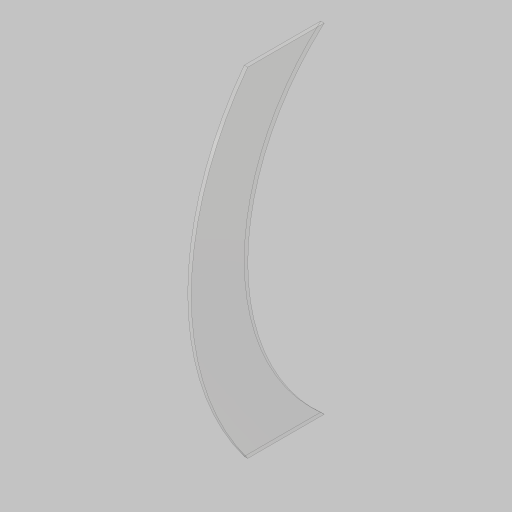
# Autodesk Inventor part: GP5-001
Saved by Autodesk Inventor 2023.5 (Build 275446000, 446)
## iProperties
Created: 2025-01-29
Part Number: GP5-001
Material: Polycarbonate, Clear
Document SubType Name: Sheet Metal
Designer: slick
Density: 1.2 g/cm^3
Sheet Metal Rule: Default
Appearance: Polycarbonate - Clear
Author: slick
Autodesk Inventor part; units mm, degrees
ref_plane "YZ Plane" through (0, 0, 0) normal (1, 0, 0) x (0, 1, 0)
ref_plane "XZ Plane" through (0, 0, 0) normal (0, 1, 0) x (-1, 0, 0)
ref_plane "XY Plane" through (0, 0, 0) normal (0, 0, 1) x (1, 0, 0)
sketch "Sketch1" plane through (0, 0, 0) normal (1, 0, 0) x (0, 1, 0)
  circle A0 centre (0, 0) radius 203.2 construction
  arc A1 (152.4, 134.4042) -> (-152.4, 134.4042) centre (0, 0) ccw
  arc A2 (152.4, 203.2) -> (-152.4, 203.2) centre (0, 0) ccw
  line L0 (152.4, 203.2) -> (152.4, 134.4042)
  line L1 (-152.4, 134.4042) -> (-152.4, 203.2)
  dimension "d0" = 406.4
  dimension "d1" = 50.8
  dimension "d2" = 152.4
  dimension "d3" = 152.4
  measures "d0" diameter of A0
  measures "d1" radial gap between concentric circles of A2 A0
  measures "d2" distance from line of A0.centre L0
  measures "d3" distance from line of A0.centre L1
extrude "Plate1" add sketch "Sketch1" along normal mid plane 3.175
equation "\"d3\" = d2"
equation "\"d4\" = Thickness"
equation "\"BendRadius\" = Thickness"
equation "\"BendReliefWidth\" = Thickness"
equation "\"BendReliefDepth\" = 0.5 * Thickness"
equation "\"CornerReliefSize\" = 4 * Thickness"
equation "\"MinimumRemnant\" = 2 * Thickness"
equation "\"TransitionRadius\" = BendRadius"
equation "\"JacobiRadiusSize\" = BendRadius"
equation "\"GapSize\" = Thickness"
equation "\"Thickness\" = 3.175"
body "Solid1"
